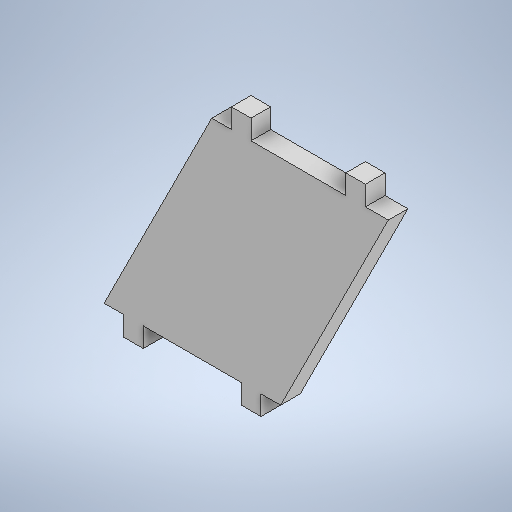
# Autodesk Inventor part: ENTRE_ASA
Saved by Autodesk Inventor 2025.1 (Build 291241000, 241)
## iProperties
Created: 2024-10-24
Part Number: ENTRE_ASA
Material: Genérico
Document SubType Name: Modeling
Designer: ambrosildo
Density: 1 g/cm^3
Appearance: Padrão
Author: ambrosildo
Autodesk Inventor part; units mm, degrees
ref_plane "YZ Plane" through (0, 0, 0) normal (1, 0, 0) x (0, 1, 0)
ref_plane "XZ Plane" through (0, 0, 0) normal (0, 1, 0) x (-1, 0, 0)
ref_plane "XY Plane" through (0, 0, 0) normal (0, 0, 1) x (1, 0, 0)
sketch "Esboço1" plane through (0, 0, 0) normal (0, 0, 1) x (1, 0, 0)
  line L0 (0, 0) -> (16.4719, 32.7528)
  line L1 (16.4719, 32.7528) -> (43.4719, 32.7528)
  line L2 (0, 0) -> (27, 0)
  line L3 (27, 0) -> (43.4719, 32.7528)
  dimension "d6" = 27
  dimension "d7" = 27
  dimension "d9" = 24.1213
  constraints: 8 end point, 1 horizontal
  measures "d6" distance of L0.end L1.end
  measures "d7" distance of L0.start L2.end
  measures "d9" distance between parallel lines of L3 L0
extrude "Extrusão1" add sketch "Esboço1" along normal blind 3
sketch "Esboço2" plane through (16.4719, 32.7528, 0) normal (0, 1, 0) x (1, 0, 0)
  line L0 (27, 0) -> (0, 0) projected
  line L1 (27, -3) -> (0, -3) projected
  line L2 (23.5, 0) -> (20.5, 0)
  line L3 (20.5, 0) -> (20.5, -3)
  line L4 (20.5, -3) -> (23.5, -3)
  line L5 (23.5, -3) -> (23.5, 0)
  line L6 (3, 0) -> (6, 0)
  line L7 (6, 0) -> (6, -3)
  line L8 (6, -3) -> (3, -3)
  line L9 (3, -3) -> (3, 0)
  point P0 (-16.4719, 0)
  dimension "d13" = 3
  dimension "d14" = 3
  dimension "d16" = 3
  dimension "d17" = 3
  constraints: 16 end point, 4 parallel, 2 horizontal, 2 perpendicular, 2 point on line
  measures "d13" distance of L4.end L3.end
  measures "d14" distance of L3.end L2.end
  measures "d16" distance of L7.end L8.end
  measures "d17" distance of L6.end L7.end
extrude "Extrusão2" add sketch "Esboço2" along normal blind 3 contours L5 L1 L3 L0 | L7 L1 L9 L0
sketch "Esboço3" plane through (0, 0, 0) normal (0, -1, 0) x (1, 0, 0)
  line L0 (16.4719, 3) -> (0, 3) projected
  line L1 (27, 0) -> (27, 3) projected
  line L2 (36.9719, 3) -> (22.4719, 3) projected
  line L3 (3, 3) -> (6, 3)
  line L4 (6, 3) -> (6, 0)
  line L5 (6, 0) -> (3, 0)
  line L6 (3, 0) -> (3, 3)
  line L7 (24, 3) -> (21, 3)
  line L8 (21, 3) -> (21, 0)
  line L9 (21, 0) -> (24, 0)
  line L10 (24, 0) -> (24, 3)
  point P0 (0, 0)
  dimension "d21" = 3
  dimension "d22" = 3
  dimension "d23" = 3
  dimension "d24" = 3
  dimension "d25" = 3
  constraints: 16 end point, 4 parallel, 2 horizontal, 2 perpendicular, 2 point on line
  measures "d21" distance of L1.end L7.start
  measures "d22" distance of L4.end L5.end
  measures "d23" distance of L3.end L4.end
  measures "d24" distance of L9.end L8.end
  measures "d25" distance of L8.end L7.end
extrude "Extrusão3" add sketch "Esboço3" along normal blind 3
